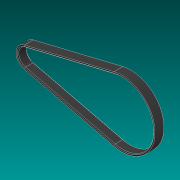
# Autodesk Inventor part: Tandriem20naar60T
Saved by Autodesk Inventor 2020.2 (Build 242310000, 310)
## iProperties
Created: 2020-05-14
Part Number: Tandriem20naar60T
Material: Rubber
Document SubType Name: Modeling
Designer: Svend
Density: 0.93 g/cm^3
Appearance: Rubber - Black
Author: Svend
Autodesk Inventor part; units mm, degrees
ref_plane "YZ Plane" through (0, 0, 0) normal (1, 0, 0) x (0, 1, 0)
ref_plane "XZ Plane" through (0, 0, 0) normal (0, 1, 0) x (-1, 0, 0)
ref_plane "XY Plane" through (0, 0, 0) normal (0, 0, 1) x (1, 0, 0)
sketch "Sketch1" plane through (0, 0, 0) normal (0, 0, 1) x (1, 0, 0)
  arc A0 (-1.4131, 5.8312) -> (-1.4131, -5.8312) centre (0, 0) ccw
  arc A1 (58.7458, -20.4093) -> (58.7458, 20.4093) centre (63.6915, 0) ccw
  line L0 (-1.4131, 5.8312) -> (58.7458, 20.4093)
  line L1 (-1.4131, -5.8312) -> (58.7458, -20.4093)
  line L2 (58.4396, 21.6727) -> (-1.7192, 7.0947)
  arc A2 (-1.7192, 7.0947) -> (-1.7192, -7.0947) centre (0, 0) ccw
  line L3 (-1.7192, -7.0947) -> (58.4396, -21.6727)
  arc A3 (58.4396, -21.6727) -> (58.4396, 21.6727) centre (63.6915, 0) ccw
  dimension "d0" = 12
  dimension "d1" = 42
  dimension "d2" = 61.9
  dimension "d3" = 1.3
  constraints: 8 end point, 8 point on circle, 4 centre point, 4 tangent, 1 coincident, 1 horizontal alignment, 3 other
  measures "d0" diameter of A0
  measures "d1" diameter of A1
  measures "d2" distance of L0.start L0.end
  measures "d3" distance between parallel lines of L0 L2
extrude "Extrusion1" add sketch "Sketch1" along normal mid plane 6
chamfer "Chamfer1" distance 0.5 angle 45 8 edges at (-6, 0, 3) (28.6664, 13.1203, 3) (84.6915, 0, 3) (28.6664, -13.1203, 3) (-6, 0, -3) (28.6664, -13.1203, -3) (84.6915, 0, -3) (28.6664, 13.1203, -3)
body "Solid1"
